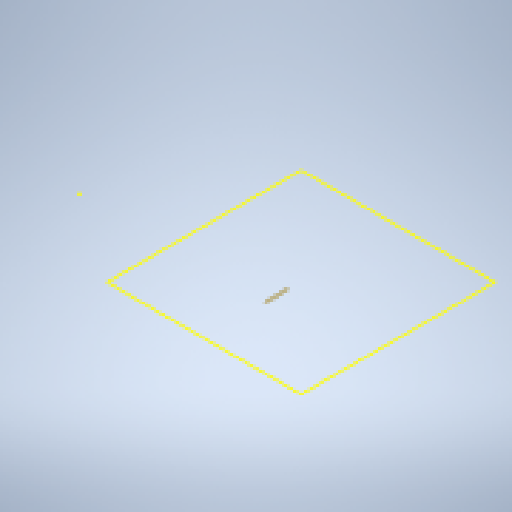
# Autodesk Inventor part: Window
Saved by Autodesk Inventor 2024 (Build 280153000, 153)
## iProperties
Created: 2023-09-11
Part Number: Window
Material: Generic
Document SubType Name: Modeling
Designer: Bruno
Density: 1 g/cm^3
Appearance: Default
Author: Bruno
Autodesk Inventor part; units mm, degrees
ref_plane "YZ Plane" through (0, 0, 0) normal (1, 0, 0) x (0, 1, 0)
ref_plane "XZ Plane" through (0, 0, 0) normal (0, 1, 0) x (-1, 0, 0)
ref_plane "XY Plane" through (0, 0, 0) normal (0, 0, 1) x (1, 0, 0)
ref_plane "Work Plane1" through (267.4086, -145.9522, -29.8619) normal (0, 1, 0) x (-1, 0, 0)
sketch "Sketch1" plane through (267.4086, -145.9522, -29.8619) normal (0, 1, 0) x (-1, 0, 0)
  line L0 (138.5, -160) -> (-141.5, -160) projected
  line L1 (138.5, 120) -> (138.5, -160) projected
  line L2 (-141.5, 120) -> (138.5, 120) projected
  line L3 (-141.5, -160) -> (-141.5, 120) projected
  point P0 (267.4086, 29.8619)
extrude "Extrusion1" add sketch "Sketch1" along normal blind 2
body "Solid1"
